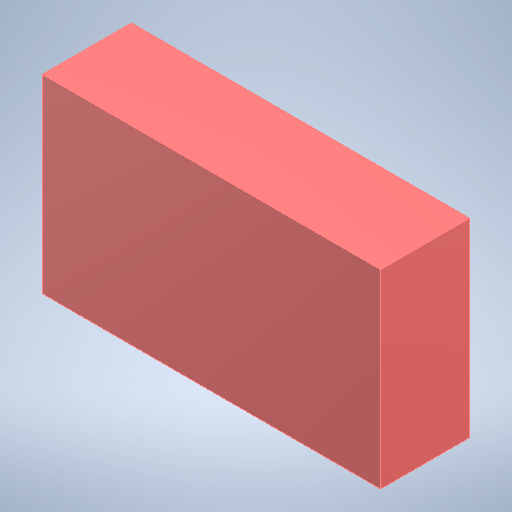
# Autodesk Inventor part: 450mah
Saved by Autodesk Inventor 2025.1 (Build 291241000, 241)
## iProperties
Created: 2024-09-04
Part Number: 450mah
Material: 一般
Document SubType Name: Modeling
Designer: right
Density: 1.86404 g/cm^3
Appearance: 滑らか - 赤
Mass: 51 g
Surface Area: 63.18 cm^2
Volume: 27.36 cm^3
Author: right
Autodesk Inventor part; units mm, degrees
ref_plane "YZ Plane" through (0, 0, 0) normal (1, 0, 0) x (0, 1, 0)
ref_plane "XZ Plane" through (0, 0, 0) normal (0, 1, 0) x (-1, 0, 0)
ref_plane "XY Plane" through (0, 0, 0) normal (0, 0, 1) x (1, 0, 0)
sketch "スケッチ1" plane through (0, 0, 0) normal (0, 0, 1) x (1, 0, 0)
  line L0 (-28.5, -16) -> (28.5, -16)
  line L1 (28.5, -16) -> (28.5, 16)
  line L2 (28.5, 16) -> (-28.5, 16)
  line L3 (-28.5, 16) -> (-28.5, -16)
  line L4 (-28.5, -16) -> (28.5, 16) construction
  line L5 (28.5, -16) -> (-28.5, 16) construction
  point P0 (0, 0)
  dimension "d0" = 57
  dimension "d1" = 32
  constraints: 12 end point, 2 midpoint, 2 parallel, 1 horizontal, 1 perpendicular
  measures "d0" distance of L2.end L1.end
  measures "d1" distance of L1.end L0.end
extrude "押し出し1" add sketch "スケッチ1" along normal blind 15
